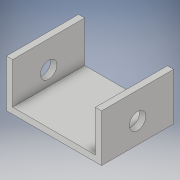
# Autodesk Inventor part: base support
Saved by Autodesk Inventor 2019 (Build 230136000, 136)
## iProperties
Created: 2021-05-25
Part Number: base support
Material: Genérico
Document SubType Name: Modeling
Designer: Juan M. Casillas
Density: 1 g/cm^3
Appearance: Valor por defecto
Author: Juan M. Casillas
Autodesk Inventor part; units mm, degrees
ref_plane "YZ Plane" through (0, 0, 0) normal (1, 0, 0) x (0, 1, 0)
ref_plane "XZ Plane" through (0, 0, 0) normal (0, 1, 0) x (-1, 0, 0)
ref_plane "XY Plane" through (0, 0, 0) normal (0, 0, 1) x (1, 0, 0)
sketch "Sketch1" plane through (0, 0, 0) normal (0, 1, 0) x (-1, 0, 0)
  line L0 (23.1, 17.5) -> (-23.1, 17.5)
  line L1 (-23.1, 17.5) -> (-23.1, -17.5)
  line L2 (-23.1, -17.5) -> (23.1, -17.5)
  line L3 (23.1, -17.5) -> (23.1, 17.5)
  line L4 (23.1, 17.5) -> (-23.1, -17.5) construction
  line L5 (-23.1, 17.5) -> (23.1, -17.5) construction
  point P0 (0, 0)
  dimension "d0" = 46.2
  dimension "d1" = 35
  constraints: 12 end point, 2 midpoint, 2 parallel, 1 horizontal, 1 perpendicular
  measures "d0" distance of L2.end L1.end
  measures "d1" distance of L1.end L0.end
extrude "Extrusion1" add sketch "Sketch1" along normal blind 3
sketch "Sketch2" plane through (0, 3, 0) normal (0, 1, 0) x (1, 0, 0)
  line L0 (-23.1, -17.5) -> (23.1, -17.5) projected
  line L1 (23.1, -17.5) -> (23.1, 17.5) projected
  line L2 (23.1, 17.5) -> (-23.1, 17.5) projected
  line L3 (-23.1, 17.5) -> (-23.1, -17.5) projected
  line L4 (-23.1, -17.5) -> (23.1, -17.5) projected
  line L5 (23.1, 17.5) -> (-23.1, 17.5) projected
  line L6 (-23.1, -17.5) -> (-20.1, -17.5)
  line L7 (-20.1, -17.5) -> (-20.1, 17.5)
  line L8 (-20.1, 17.5) -> (-23.1, 17.5)
  line L9 (-23.1, 17.5) -> (-23.1, -17.5)
  line L10 (23.1, -17.5) -> (20.1, -17.5)
  line L11 (20.1, -17.5) -> (20.1, 17.5)
  line L12 (20.1, 17.5) -> (23.1, 17.5)
  line L13 (23.1, 17.5) -> (23.1, -17.5)
  point P0 (0, 0)
  dimension "d4" = 3
  dimension "d5" = 3
  constraints: 16 end point, 4 parallel, 2 horizontal, 2 perpendicular, 2 point on line
  measures "d4" distance of L8.end L7.end
  measures "d5" distance of L11.end L12.end
extrude "Extrusion2" add sketch "Sketch2" along normal blind 20 contours L3 L2 L7 L0 | L11 L2 L1 L0
sketch "Sketch3" plane through (23.1, 0, 17.5) normal (1, 0, 0) x (0, 0, -1)
  line L0 (0, 0) -> (35, 0) construction
  line L1 (35, 0) -> (35, 23) construction
  line L2 (0, 23) -> (35, 23) construction
  line L3 (0, 0) -> (0, 23) construction
  line L4 (0, 23) -> (35, 23) construction
  line L5 (17.5, 23) -> (17.5, 0) construction
  line L6 (17.5, 0) -> (17.5, 10) construction
  circle A0 centre (17.5, 10) radius 4
  dimension "d8" = 10
  dimension "d9" = 8
  constraints: 4 end point, 1 centre point, 1 coincident, 1 midpoint, 1 point on line, 1 vertical
  measures "d8" distance of L5.end L6.end
  measures "d9" diameter of A0
extrude "Extrusion3" cut sketch "Sketch3" against normal through all
body "Solid1"
